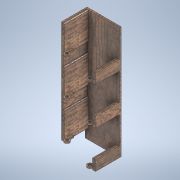
# Autodesk Inventor part: Interior Der
Saved by Autodesk Inventor 2021 (Build 250183000, 183)
## iProperties
Created: 2021-06-27
Part Number: Interior Der
Material: Plástico PBT
Document SubType Name: Modeling
Designer: artur
Density: 1.31 g/cm^3
Appearance: Fresno blanco - Java
Mass: 509.351 g
Surface Area: 1561.21 cm^2
Volume: 388.818 cm^3
Author: artur
Autodesk Inventor part; units mm, degrees
sketch "Boceto1" plane through (0, 0, 0) normal (1, 0, 0) x (0, 1, 0)
  line L0 (0, 0) -> (330, 0)
  line L1 (330, 0) -> (330, -75)
  line L2 (330, -75) -> (0, -75)
  line L3 (0, -75) -> (0, 0)
  dimension "d0" = 330
  dimension "d1" = 75
  constraints: 8 end point, 2 parallel, 1 horizontal, 1 perpendicular
  measures "d0" distance of L1.end L2.end
  measures "d1" distance of L0.end L1.end
extrude "Extrusión1" add sketch "Boceto1" along normal blind 5
sketch "Boceto2" plane through (5, 0, 0) normal (1, 0, 0) x (0, 0, -1)
  line L0 (75, 330) -> (0, 330) projected
  line L1 (75, 0) -> (75, 330) projected
  line L2 (0, 330) -> (75, 330)
  line L3 (75, 330) -> (75, 250)
  line L4 (75, 250) -> (0, 250)
  line L5 (0, 250) -> (0, 330)
  line L6 (75, 140) -> (0, 140)
  line L7 (0, 140) -> (0, 220)
  line L8 (0, 220) -> (75, 220)
  line L9 (75, 220) -> (75, 140)
  line L10 (75, 30) -> (0, 30)
  line L11 (0, 30) -> (0, 110)
  line L12 (0, 110) -> (75, 110)
  line L13 (75, 110) -> (75, 30)
  point P0 (0, 0)
  dimension "d4" = 80
  dimension "d7" = 110
  constraints: 24 end point, 2 parallel, 1 horizontal, 1 perpendicular, 1 point on line, 1 vertical, 16 other
  measures "d4" distance between parallel lines of L4 L0
  measures "d7" distance of L3.end L6.start
extrude "Extrusión2" add sketch "Boceto2" along normal blind 4
sketch "Boceto3" plane through (0, 330, 0) normal (0, 1, 0) x (1, 0, 0)
  line L0 (7, 0) -> (4, 0)
  line L1 (4, 0) -> (4, 75)
  line L2 (4, 75) -> (7, 75)
  line L3 (7, 75) -> (7, 0)
  line L4 (0, 75) -> (0, 0) projected
  line L5 (9, 75) -> (9, 0) projected
  line L6 (0, 0) -> (9, 0) projected
  line L7 (0, 75) -> (9, 75) projected
  dimension "d14" = 4
  dimension "d15" = 2
  dimension "d16" = 0
  dimension "d17" = 0
  dimension "d62" = 3
  constraints: 8 end point, 2 parallel, 1 horizontal, 1 perpendicular
  measures "d14" distance between parallel lines of L4 L1
  measures "d15" distance between parallel lines of L3 L5
  measures "d16" distance between parallel lines of L6 L0
  measures "d17" distance between parallel lines of L7 L2
  measures "d62" distance between parallel lines of L1 L3
sketch "Boceto8" plane through (5, 220, 0) normal (0, 1, 0) x (1, 0, 0)
  line L0 (-1, 0) -> (-1, 75) projected
  line L1 (2, 75) -> (2, 0) projected
  line L2 (-5, 0) -> (4, 0) projected
  line L3 (-5, 75) -> (4, 75) projected
sketch "Boceto9" plane through (5, 110, 0) normal (0, 1, 0) x (1, 0, 0)
  line L0 (2, 75) -> (2, 0) projected
  line L1 (-1, 0) -> (-1, 75) projected
  line L2 (-5, 0) -> (4, 0) projected
  line L3 (-5, 75) -> (4, 75) projected
extrude "Extrusión3" cut sketch "Boceto3" against normal blind 30 contours L0 L1 L2 L3
extrude "Extrusión4" cut sketch "Boceto8" against normal blind 30
extrude "Extrusión5" cut sketch "Boceto9" against normal blind 30
sketch "Boceto10" plane through (0, 0, 0) normal (-1, 0, 0) x (0, 0, 1)
  line L0 (-75, 0) -> (-75, 330) projected
  line L1 (-75, 330) -> (0, 330) projected
  line L2 (-75, 0) -> (-70, 0)
  line L3 (-70, 0) -> (-70, 330)
  line L4 (-70, 330) -> (-75, 330)
  line L5 (-75, 330) -> (-75, 0)
  point P0 (0, 0)
  dimension "d24" = 5
  constraints: 8 end point, 2 parallel, 1 horizontal, 1 perpendicular, 1 point on line
  measures "d24" distance between parallel lines of L0 L3
extrude "Extrusión6" add sketch "Boceto10" against normal blind 100
sketch "Boceto11" plane through (5, 0, -70) normal (0, 0, 1) x (1, 0, 0)
  line L0 (95, 330) -> (95, 0) projected
  line L1 (-5, 0) -> (95, 0) projected
  line L2 (95, 330) -> (90, 330)
  line L3 (90, 330) -> (90, 0)
  line L4 (90, 0) -> (95, 0)
  line L5 (95, 0) -> (95, 330)
  dimension "d27" = 5
  constraints: 8 end point, 2 parallel, 1 horizontal, 1 perpendicular, 1 point on line
  measures "d27" distance between parallel lines of L3 L0
extrude "Extrusión7" add sketch "Boceto11" along normal blind 70
sketch "Boceto12" plane through (95, 0, -70) normal (-1, 0, 0) x (0, 0, 1)
  line L0 (70, 0) -> (70, 330) projected
  line L1 (-5, 0) -> (-5, 330) projected
  line L2 (70, 250) -> (-5, 250)
  line L3 (-5, 250) -> (-5, 220)
  line L4 (-5, 220) -> (70, 220)
  line L5 (70, 220) -> (70, 250)
  line L6 (-5, 330) -> (70, 330) projected
  line L7 (70, 140) -> (-5, 140)
  line L8 (-5, 140) -> (-5, 110)
  line L9 (-5, 110) -> (70, 110)
  line L10 (70, 110) -> (70, 140)
  line L11 (70, 30) -> (-5, 30)
  line L12 (-5, 30) -> (-5, 0)
  line L13 (-5, 0) -> (70, 0)
  line L14 (70, 0) -> (70, 30)
  point P0 (70, 0)
  point P1 (70, 30)
  point P2 (-5, 30)
  point P3 (70, 140)
  point P4 (-5, 140)
  point P5 (-5, 250)
  dimension "d30" = 80
  dimension "d31" = 30
  dimension "d34" = 110
  constraints: 24 end point, 2 parallel, 2 point on line, 1 horizontal, 1 perpendicular, 1 vertical, 16 other
  measures "d30" distance between parallel lines of L6 L2
  measures "d31" distance between parallel lines of L2 L4
  measures "d34" distance of L2.start L7.start
extrude "Extrusión8" add sketch "Boceto12" along normal blind 4 contours L13 L1 L11 L0 | L9 L1 L7 L0 | L4 L1 L2 L0
sketch "Boceto16" plane through (100, 0, 0) normal (1, 0, 0) x (0, 0, -1)
  line L0 (70, 250) -> (0, 250) projected
  line L1 (0, 330) -> (0, 250) projected
  line L2 (70, 330) -> (0, 330) projected
  line L3 (70, 250) -> (70, 330) projected
  line L4 (70, 140) -> (0, 140) projected
  line L5 (0, 220) -> (0, 140) projected
  line L6 (0, 220) -> (70, 220) projected
  line L7 (70, 140) -> (70, 220) projected
  line L8 (70, 30) -> (0, 30) projected
  line L9 (0, 110) -> (0, 30) projected
  line L10 (0, 110) -> (70, 110) projected
  line L11 (70, 30) -> (70, 110) projected
  point P0 (0, 0)
extrude "Extrusión12" cut sketch "Boceto16" against normal blind 10
sketch "Boceto25" plane through (0, 0, 0) normal (0, 0, 1) x (1, 0, 0)
  line L0 (7, 330) -> (7, 300) construction
  line L1 (7, 300) -> (7, 330) construction
  line L2 (7, 330) -> (125.2499, 220) construction
  line L3 (7, 330) -> (9, 328.1395)
  line L4 (9, 330) -> (9, 250) projected
  line L5 (7, 330) -> (9, 330) projected
  line L6 (8, 330) -> (7, 330)
  line L7 (7, 220) -> (9, 220) projected
  line L8 (7, 220) -> (9, 218.1395)
  line L9 (9, 220) -> (9, 140) projected
  line L10 (7, 220) -> (9.7315, 220) construction
  line L11 (9, 218.1395) -> (9, 220)
  line L12 (9, 220) -> (7, 220)
  line L13 (7, 110) -> (9, 110) projected
  line L14 (7, 110) -> (9, 108.1395)
  line L15 (9, 108.1395) -> (9, 110)
  line L16 (9, 110) -> (7, 110)
  point P0 (0, 0)
  dimension "d57" = 42.93
  dimension "d106" = 42.93
  constraints: 22 end point, 5 point on line, 3 perpendicular, 2 collinear, 2 horizontal, 1 equal length, 1 parallel
  measures "d57" angle of L8 L10
  measures "d106" angle of L3 L6
extrude "Extrusión13" cut sketch "Boceto25" against normal blind 70
sketch "Boceto26" plane through (5, 0, 0) normal (1, 0, 0) x (0, 0, -1)
  line L0 (70, 0) -> (70, 30) projected
  line L1 (70, 30) -> (0, 30) projected
  line L2 (0, 30) -> (0, 0) projected
  line L3 (0, 0) -> (70, 0) projected
extrude "Extrusión14" cut sketch "Boceto26" against normal blind 10
sketch "Boceto27" plane through (91, 220, -70) normal (0, -1, 0) x (1, 0, 0)
  line L0 (0, 0) -> (0, 70) construction
  line L1 (0, 70) -> (-37.4235, 70) construction
  circle A0 centre (-7.5, 70) radius 7.5
  line L2 (0, 50) -> (-7.5, 50)
  line L3 (-7.5, 50) -> (-7.5, 70)
  line L4 (-7.5, 70) -> (0, 70)
  line L5 (0, 70) -> (0, 50)
  circle A1 centre (-7.5, 70) radius 4
  point P0 (-91, 70)
  point P1 (-7.5, 62.5)
  dimension "d64" = 15
  dimension "d63" = 20
  dimension "d65" = 8
  constraints: 10 end point, 2 horizontal, 2 parallel, 2 point on line, 1 centre point, 1 coincident, 1 perpendicular, 3 other
  measures "d63" distance of L2.end L3.end
  measures "d65" diameter of A1
sketch "Boceto28" plane through (91, 110, -70) normal (0, -1, 0) x (1, 0, 0)
  line L0 (0, 50) -> (-7.5, 50) projected
  line L1 (-7.5, 50) -> (-7.5, 70) projected
  circle A0 centre (-7.5, 70) radius 7.5 projected
  circle A1 centre (-7.5, 70) radius 4 projected
  line L2 (0, 70) -> (-37.4235, 70) construction
  line L3 (0, 70) -> (0, 50) projected
  point P0 (-91, 70)
  point P1 (-7.5, 62.5)
sketch "Boceto29" plane through (0, 0, -75) normal (0, -1, 0) x (1, 0, 0)
  line L0 (91, 55) -> (83.5, 55) projected
  line L1 (83.5, 55) -> (83.5, 75) projected
  circle A0 centre (83.5, 75) radius 7.5 projected
  circle A1 centre (83.5, 75) radius 4 projected
  line L2 (83.5, 75) -> (91, 75) projected
  line L3 (91, 75) -> (91, 55) projected
  point P0 (0, 75)
  point P1 (83.5, 67.5)
extrude "Extrusión15" add sketch "Boceto27" against normal blind 8.4 contours L4 A1 L3 A0 | L5 L2 L3 A0 | A0 L3 A1 L4
extrude "Extrusión16" add sketch "Boceto28" against normal blind 8.4
extrude "Extrusión17" add sketch "Boceto29" against normal blind 8.4 contours L0 L1 A0 L3 | L2 A1 L1 A0 | A0 L1 A1 L2
sketch "Boceto30" plane through (91, 220, -70) normal (0, -1, 0) x (1, 0, 0)
  circle A0 centre (-7.5, 70) radius 4 projected
  line L0 (0, 0) -> (-91, 0) projected
  line L1 (-91, 0) -> (-91, -5) projected
  line L2 (-91, -5) -> (9, -5) projected
  line L3 (9, -5) -> (9, 70) projected
  line L4 (9, 70) -> (0, 70) projected
  arc A1 (0, 70) -> (-7.5, 62.5) centre (-7.5, 70) ccw projected
  line L5 (-7.5, 62.5) -> (-7.5, 50) projected
  line L6 (-7.5, 50) -> (0, 50) projected
  line L7 (0, 0) -> (0, 50) projected
  line L8 (0, 50) -> (0, 70)
  point P0 (-91, 70)
  constraints: 2 end point
sketch "Boceto31" plane through (91, 110, -70) normal (0, -1, 0) x (1, 0, 0)
  line L0 (0, 50) -> (0, 70) projected
  circle A0 centre (-7.5, 70) radius 4 projected
  line L1 (9, 0) -> (0, 0) projected
  line L2 (9, 70) -> (9, 0) projected
  line L3 (0, 70) -> (9, 70) projected
  arc A1 (0, 70) -> (-7.5, 62.5) centre (-7.5, 70) ccw projected
  line L4 (-7.5, 62.5) -> (-7.5, 50) projected
  line L5 (-7.5, 50) -> (0, 50) projected
  line L6 (0, 0) -> (0, 50) projected
  point P0 (-91, 70)
sketch "Boceto32" plane through (0, 0, -75) normal (0, -1, 0) x (1, 0, 0)
  circle A0 centre (83.5, 75) radius 4 projected
  line L0 (100, 5) -> (91, 5) projected
  line L1 (100, 75) -> (100, 5) projected
  line L2 (91, 75) -> (100, 75) projected
  arc A1 (91, 75) -> (83.5, 67.5) centre (83.5, 75) ccw projected
  line L3 (83.5, 67.5) -> (83.5, 55) projected
  line L4 (83.5, 55) -> (91, 55) projected
  line L5 (91, 5) -> (91, 55) projected
  line L6 (91, 55) -> (91, 75) projected
  point P0 (0, 75)
extrude "Extrusión18" cut sketch "Boceto32" against normal blind 4.2 contours L4 L3 A1 L6
extrude "Extrusión19" cut sketch "Boceto31" against normal blind 4.2 contours L5 L4 A1 L0
extrude "Extrusión20" cut sketch "Boceto30" against normal blind 4.2 contours L6 L5 A1 L8
thread "Rosca1" size "M8x1.25" class "6H" standard "ANSI Metric M Profile" full length
ref_plane "Work Plane2" through (5, 254.2, 0) normal (0, -1, 0) x (1, 0, 0)
sketch "Sketch33" plane through (5, 254.2, 0) normal (0, -1, 0) x (1, 0, 0)
  line L0 (4, 0) -> (4, -20)
  line L1 (4, -20) -> (11.5, -20)
  line L2 (11.5, -20) -> (11.5, 0)
  line L3 (11.5, 0) -> (4, 0)
  circle A0 centre (11.5, 0) radius 4
  circle A1 centre (11.5, 0) radius 7.5
  point P0 (-5, 0)
  point P1 (4, 0)
  point P2 (11.5, -7.5)
  dimension "d81" = 20
  dimension "d82" = 7.5
  dimension "d83" = 20
  dimension "d84" = 8
  dimension "d85" = 15
  constraints: 8 end point, 2 centre point, 2 coincident, 2 perpendicular, 1 vertical
  measures "d81" distance of L0.start L0.end
  measures "d82" distance of L0.end L1.end
  measures "d83" distance of L1.end L2.end
  measures "d84" diameter of A0
  measures "d85" diameter of A1
extrude "Extrusion21" add sketch "Sketch33" against normal blind 4.2 contours A1 L2 L1 L0 | A1 L2 A0 L3 | L3 A0 L2 A1
ref_plane "Work Plane3" through (5, 144.2, 0) normal (0, -1, 0) x (1, 0, 0)
sketch "Sketch34" plane through (5, 144.2, 0) normal (0, -1, 0) x (1, 0, 0)
  line L0 (4, 0) -> (4, -20)
  line L1 (4, -20) -> (11.5, -20)
  line L2 (11.5, -20) -> (11.5, 0)
  line L3 (11.5, 0) -> (4, 0)
  circle A0 centre (11.5, 0) radius 4
  circle A1 centre (11.5, 0) radius 7.5
  point P0 (-5, 0)
  point P1 (11.5, -7.5)
  dimension "d89" = 20
  dimension "d90" = 7.5
  dimension "d91" = 20
  dimension "d92" = 8
  dimension "d93" = 15
  constraints: 8 end point, 2 centre point, 2 coincident, 2 perpendicular, 1 vertical
  measures "d89" distance of L0.start L0.end
  measures "d90" distance of L0.end L1.end
  measures "d91" distance of L1.end L2.end
  measures "d92" diameter of A0
  measures "d93" diameter of A1
extrude "Extrusion22" add sketch "Sketch34" against normal blind 4.2 contours A1 L2 L1 L0 | A1 L2 A0 L3 | L3 A0 L2 A1
ref_plane "Work Plane4" through (0, 34.2, 0) normal (0, -1, 0) x (1, 0, 0)
sketch "Sketch35" plane through (0, 34.2, 0) normal (0, -1, 0) x (1, 0, 0)
  line L0 (9, 0) -> (9, -20)
  line L1 (9, -20) -> (16.5, -20)
  line L2 (16.5, -20) -> (16.5, 0)
  line L3 (16.5, 0) -> (9, 0)
  circle A0 centre (16.5, 0) radius 4
  circle A1 centre (16.5, 0) radius 7.5
  point P0 (0, 0)
  point P1 (9, 0)
  point P2 (16.5, -7.5)
  dimension "d97" = 20
  dimension "d98" = 7.5
  dimension "d99" = 20
  dimension "d100" = 8
  dimension "d101" = 15
  constraints: 8 end point, 2 centre point, 2 coincident, 2 perpendicular, 1 vertical
  measures "d97" distance of L0.start L0.end
  measures "d98" distance of L0.end L1.end
  measures "d99" distance of L1.end L2.end
  measures "d100" diameter of A0
  measures "d101" diameter of A1
extrude "Extrusion23" add sketch "Sketch35" against normal blind 4.2 contours A1 L2 L1 L0 | A1 L2 A0 L3 | L3 A0 L2 A1
thread "Thread2" size "M8x1.25" class "6H" standard "ANSI Metric M Profile" full length
sketch "Boceto13" plane through (95, 250, 0) normal (0, 1, 0) x (1, 0, 0)
  line L0 (5, 70) -> (-4, 70) projected
  line L1 (-4, 0) -> (5, 0) projected
  line L2 (-2, 70) -> (1, 70)
  line L3 (1, 70) -> (1, 0)
  line L4 (1, 0) -> (-2, 0)
  line L5 (-2, 0) -> (-2, 70)
  line L6 (-4, 0) -> (-4, 70) projected
  point P0 (-2, 0)
  point P1 (1, 70)
  dimension "d113" = 2
  dimension "d114" = 3
  constraints: 8 end point, 2 parallel, 2 point on line, 1 horizontal, 1 perpendicular
  measures "d113" distance between parallel lines of L6 L5
  measures "d114" distance between parallel lines of L3 L5
extrude "Extrusión24" cut sketch "Boceto13" against normal blind 20 contours L3 L1 L5 L0
pattern_linear "Patrón rectangular1" count 3 spacing 110 along (0, -1, 0) of "Extrusión24"
equation "\"d57\" = d106"
